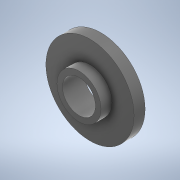
# Autodesk Inventor part: L3040-8110TB
Saved by Autodesk Inventor 2020 (Build 240168000, 168)
## iProperties
Part Number: L3040-8110TB
Material: アルミニウム 2014-T4
Document SubType Name: Modeling
Designer: Masato Kubotera
Density: 2.8 g/cm^3
Appearance: 滑らか - 黒
Catalog Web Link: https://www.hirosugi-net.co.jp/shop/g/g103787/
Author: Masato Kubotera
Autodesk Inventor part; units mm, degrees
ref_plane "YZ Plane" through (0, 0, 0) normal (1, 0, 0) x (0, 1, 0)
ref_plane "XZ Plane" through (0, 0, 0) normal (0, 1, 0) x (-1, 0, 0)
ref_plane "XY Plane" through (0, 0, 0) normal (0, 0, 1) x (1, 0, 0)
sketch "スケッチ1" plane through (0, 0, 0) normal (0, 1, 0) x (-1, 0, 0)
  line L0 (-1.5, 0) -> (-4, 0)
  line L1 (-4, 0) -> (-4, 1)
  line L2 (-4, 1) -> (-2, 1)
  line L3 (-2, 1) -> (-2, 2)
  line L4 (-2, 2) -> (-1.5, 2)
  line L5 (0, 2) -> (0, 0) construction
  line L6 (-1.5, 2) -> (-1.5, 0)
  dimension "d0" = 1
  dimension "d1" = 8
  dimension "d2" = 1
  dimension "d3" = 3
  dimension "d4" = 4
  constraints: 14 end point, 6 perpendicular, 2 point on line, 1 horizontal
  measures "d0" distance of L0.end L1.end
  measures "d1" diameter of L1 L5
  measures "d2" distance of L2.end L3.end
  measures "d3" diameter of L6 L5
  measures "d4" diameter of L3 L5
revolve "回転1" add sketch "スケッチ1" angle 360 about axis through (0, 0, 2) along (0, 0, -1)
